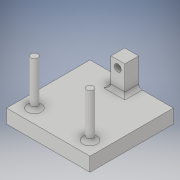
# Autodesk Inventor part: Cupholder
Saved by Autodesk Inventor 2018 (Build 220112000, 112)
## iProperties
Created: 2018-09-22
Part Number: Cupholder
Material: Generic
Document SubType Name: Modeling
Designer: Aditya Kendre
Density: 1 g/cm^3
Appearance: Default
Author: Aditya Kendre
Autodesk Inventor part; units mm, degrees
ref_plane "YZ Plane" through (0, 0, 0) normal (1, 0, 0) x (0, 1, 0)
ref_plane "XZ Plane" through (0, 0, 0) normal (0, 1, 0) x (-1, 0, 0)
ref_plane "XY Plane" through (0, 0, 0) normal (0, 0, 1) x (1, 0, 0)
sketch "Sketch1" plane through (0, 0, 0) normal (0, 1, 0) x (-1, 0, 0)
  line L0 (0, 0) -> (76.2, 0)
  line L1 (76.2, 0) -> (76.2, -76.2)
  line L2 (76.2, -76.2) -> (0, -76.2)
  line L3 (0, -76.2) -> (0, 0)
  dimension "d0" = 76.2
  dimension "d1" = 76.2
  constraints: 8 end point, 2 parallel, 1 horizontal, 1 perpendicular
  measures "d0" distance of L1.end L2.end
  measures "d1" distance of L0.end L1.end
extrude "Extrusion1" add sketch "Sketch1" along normal blind 12.7
sketch "Sketch2" plane through (0, 12.7, 0) normal (0, 1, 0) x (1, 0, 0)
  point P0 (0, 0)
  point P1 (-12.7, 12.7)
  point P2 (-63.5, 12.7)
hole "Hole1" at (-12.7, 12.7, -12.7) at (-63.5, 12.7, -12.7) direction (0, -1, 0) diameter 5.08 depth 9.525 tip angle 118
sketch "Sketch3" plane through (0, 12.7, 0) normal (0, 1, 0) x (1, 0, 0)
  line L0 (0, 76.2) -> (-76.2, 76.2) projected
  line L1 (-44.45, 76.2) -> (-31.75, 76.2)
  line L2 (-31.75, 76.2) -> (-31.75, 63.5)
  line L3 (-31.75, 63.5) -> (-44.45, 63.5)
  line L4 (-44.45, 63.5) -> (-44.45, 76.2)
  point P0 (0, 0)
  point P1 (-38.1, 76.2)
  dimension "d11" = 12.7
  dimension "d12" = 12.7
  constraints: 8 end point, 2 parallel, 1 horizontal, 1 midpoint, 1 perpendicular, 1 point on line
  measures "d11" distance of L2.end L3.end
  measures "d12" distance of L1.end L2.end
extrude "Extrusion2" add sketch "Sketch3" along normal blind 25.4
sketch "Sketch4" plane through (0, 0, -76.2) normal (0, 0, -1) x (-1, 0, 0)
  point P0 (0, 0)
  point P1 (38.1, 31.75)
hole "Hole2" at (-38.1, 31.75, -76.2) direction (0, 0, 1) diameter 6.35 depth 14.2875 tip angle 118
fillet "Fillet1" radius 3.175 3 edges at (-31.75, 12.7, -69.85) (-38.1, 12.7, -63.5) (-44.45, 12.7, -69.85)
sketch "Sketch5" plane through (0, 12.7, 0) normal (0, 1, 0) x (1, 0, 0)
  circle A0 centre (-63.5, 12.7) radius 2.54 projected
  point P0 (0, 0)
  point P1 (-12.7, 12.7)
  constraints: 1 coincident
hole "Hole3" at (-63.5, 12.7, -12.7) at (-12.7, 12.7, -12.7) direction (0, -1, 0) diameter 6.35 depth 9.525 tip angle 118
sketch "Sketch6" plane through (0, 12.7, 0) normal (0, 1, 0) x (1, 0, 0)
  circle A0 centre (-63.5, 12.7) radius 3.175 projected
  circle A1 centre (-12.6652, 12.7) radius 3.2098
  circle A2 centre (-63.5, 12.7) radius 3.175
  point P0 (0, 0)
  constraints: 3 coincident, 2 centre point, 1 concentric
extrude "Extrusion3" add sketch "Sketch6" along normal blind 41.275 and the other way blind 12.7127
fillet "Fillet2" radius 3.175 1 edges at (-15.875, 12.7, -12.7)
fillet "Fillet3" radius 3.175 1 edges at (-66.675, 12.7, -12.7)
body "Solid1"
